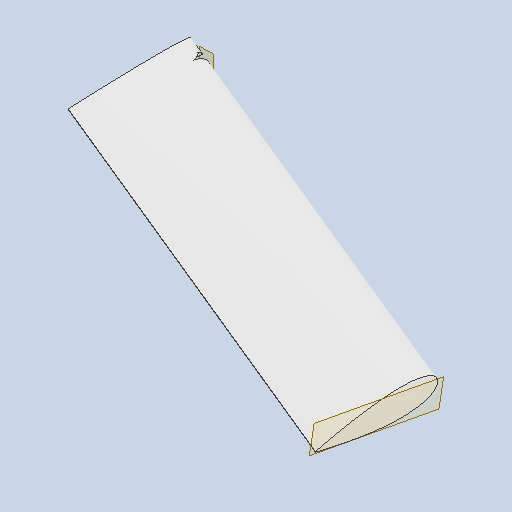
# Autodesk Inventor part: TailRight
Saved by Autodesk Inventor 2026 (Build 300175050, 175E)
## iProperties
Created: 2025-08-03
Part Number: TailRight
Material: Plastic, Opaque White
Document SubType Name: Modeling
Designer: Cupri
Density: 0.952 g/cm^3
Appearance: Smooth - White
Mass: 2293.42 g
Surface Area: 2244.69 cm^2
Volume: 2409.06 cm^3
Author: Cupri
Autodesk Inventor part; units mm, degrees
ref_plane "YZ Plane" through (0, 0, 0) normal (1, 0, 0) x (0, 1, 0)
ref_plane "XZ Plane" through (0, 0, 0) normal (0, 1, 0) x (-1, 0, 0)
ref_plane "XY Plane" through (0, 0, 0) normal (0, 0, 1) x (1, 0, 0)
sketch "Sketch1" plane through (0, 0, 0) normal (0, 0, 1) x (1, 0, 0)
  line L0 (10.5804, 9.5) -> (10.5804, 4.5) projected
  arc A0 (10.5804, 9.5) -> (10.0804, 10) centre (10.0804, 9.5) ccw projected
  line L1 (5.0804, 10) -> (10.0804, 10) projected
  line L2 (3.5804, 8.5) -> (5.0804, 10) projected
  line L3 (6.7804, 8.5) -> (3.5804, 8.5) projected
  line L4 (6.7804, 7.0485) -> (6.7804, 8.5) projected
  line L5 (3.3319, 3.6) -> (6.7804, 7.0485) projected
  line L6 (-2.1711, 3.6) -> (3.3319, 3.6) projected
  line L7 (-5.6196, 7.0485) -> (-2.1711, 3.6) projected
  line L8 (-5.6196, 8.5) -> (-5.6196, 7.0485) projected
  line L9 (-2.4196, 8.5) -> (-5.6196, 8.5) projected
  line L10 (-3.9196, 10) -> (-2.4196, 8.5) projected
  line L11 (-8.9196, 10) -> (-3.9196, 10) projected
  arc A1 (-8.9196, 10) -> (-9.4196, 9.5) centre (-8.9196, 9.5) ccw projected
  line L12 (-9.4196, 4.5) -> (-9.4196, 9.5) projected
  line L13 (-7.9196, 3) -> (-9.4196, 4.5) projected
  line L14 (-7.9196, 6.2) -> (-7.9196, 3) projected
  line L15 (-6.4681, 6.2) -> (-7.9196, 6.2) projected
  line L16 (-3.0196, 2.7515) -> (-6.4681, 6.2) projected
  line L17 (-3.0196, -2.7515) -> (-3.0196, 2.7515) projected
  line L18 (-6.4681, -6.2) -> (-3.0196, -2.7515) projected
  line L19 (-7.9196, -6.2) -> (-6.4681, -6.2) projected
  line L20 (-7.9196, -3) -> (-7.9196, -6.2) projected
  line L21 (-9.4196, -4.5) -> (-7.9196, -3) projected
  line L22 (-9.4196, -9.5) -> (-9.4196, -4.5) projected
  arc A2 (-9.4196, -9.5) -> (-8.9196, -10) centre (-8.9196, -9.5) ccw projected
  line L23 (-3.9196, -10) -> (-8.9196, -10) projected
  line L24 (-2.4196, -8.5) -> (-3.9196, -10) projected
  line L25 (-5.6196, -8.5) -> (-2.4196, -8.5) projected
  line L26 (-5.6196, -7.0485) -> (-5.6196, -8.5) projected
  line L27 (-2.1711, -3.6) -> (-5.6196, -7.0485) projected
  line L28 (3.3319, -3.6) -> (-2.1711, -3.6) projected
  line L29 (6.7804, -7.0485) -> (3.3319, -3.6) projected
  line L30 (6.7804, -8.5) -> (6.7804, -7.0485) projected
  line L31 (3.5804, -8.5) -> (6.7804, -8.5) projected
  line L32 (5.0804, -10) -> (3.5804, -8.5) projected
  line L33 (10.0804, -10) -> (5.0804, -10) projected
  arc A3 (10.0804, -10) -> (10.5804, -9.5) centre (10.0804, -9.5) ccw projected
  line L34 (10.5804, -4.5) -> (10.5804, -9.5) projected
  line L35 (9.0804, -3) -> (10.5804, -4.5) projected
  line L36 (9.0804, -6.2) -> (9.0804, -3) projected
  line L37 (7.6289, -6.2) -> (9.0804, -6.2) projected
  line L38 (4.1804, -2.7515) -> (7.6289, -6.2) projected
  line L39 (4.1804, 2.7515) -> (4.1804, -2.7515) projected
  line L40 (7.6289, 6.2) -> (4.1804, 2.7515) projected
  line L41 (9.0804, 6.2) -> (7.6289, 6.2) projected
  line L42 (9.0804, 3) -> (9.0804, 6.2) projected
  line L43 (10.5804, 4.5) -> (9.0804, 3) projected
  circle A4 centre (0.5804, 0) radius 2 projected
  line L44 (-10.125, 10.125) -> (10.125, 10.125) projected
  line L45 (-10.125, -10.125) -> (-10.125, 10.125) projected
  line L46 (385, 60.6857) -> (385, -334.3432)
  line L47 (-10.125, 10.125) -> (385, -266.5445)
  line L48 (-10.125, 10.125) -> (472.2336, 10.125) construction
  line L49 (-10.125, 10.125) -> (-18.3165, 15.8608)
  line L50 (780.125, 10.125) -> (385, -266.5445)
  ellipse E0 centre (381.713, 63.1894) end of major axis (413.2942, 37.7545) minor radius 40.5498 projected
  point P0 (0, 0)
  dimension "d0" = 35
  dimension "d1" = 10
  constraints: 10 end point, 2 point on line, 1 equal length, 1 horizontal, 1 symmetric about line, 1 vertical
  measures "d0" angle of L47 L48
  measures "d1" distance of L44.start L49.end
ref_plane "Work Plane1" through (-18.3165, 15.8608, 0) normal (-0.819152, 0.5735764, 0) x (-0.5735764, -0.819152, 0)
sketch "Sketch2" plane through (-18.3165, 15.8608, 0) normal (-0.819152, 0.5735764, 0) x (-0.5735764, -0.819152, 0)
  spline S0 degree 4 poles (3.0051, 134.0148) (3.0202, 133.9433) (3.0935, 133.5946) (3.2162, 133.0098) (3.4218, 132.0236) (3.6365, 130.9884) (3.8977, 129.7198) (4.2019, 128.23) (4.5479, 126.5185) (4.9334, 124.5915) (5.356, 122.4525) (5.8134, 120.1071) (6.3027, 117.5605) (6.8216, 114.8187) (7.367, 111.8882) (7.9363, 108.7758) (8.5263, 105.4888) (9.1344, 102.0348) (9.7573, 98.422) (10.3924, 94.6587) (11.0362, 90.7538) (11.686, 86.7164) (12.3385, 82.5558) (12.9906, 78.282) (13.6392, 73.9047) (14.2807, 69.4343) (14.912, 64.8811) (15.5296, 60.2559) (16.1298, 55.5693) (16.7091, 50.8325) (17.2636, 46.0563) (17.7897, 41.252) (18.2834, 36.4308) (18.7408, 31.6039) (19.1581, 26.7826) (19.5314, 21.9782) (19.8569, 17.2018) (20.1309, 12.4646) (20.3499, 7.7777) (20.5107, 3.1519) (20.6103, -1.4019) (20.646, -5.8731) (20.6155, -10.2512) (20.5168, -14.5261) (20.3486, -18.6878) (20.1098, -22.7266) (19.8, -26.633) (19.4191, -30.3981) (18.9678, -34.0129) (18.447, -37.4692) (17.8584, -40.7589) (17.2038, -43.8744) (16.4855, -46.8085) (15.7065, -49.5545) (14.8694, -52.1063) (13.9776, -54.4581) (13.0341, -56.6048) (12.0421, -58.5418) (11.0046, -60.2651) (9.9239, -61.7712) (8.8021, -63.0569) (7.64, -64.1189) (6.4386, -64.9533) (5.1984, -65.5542) (3.9272, -65.9158) (2.6271, -66.0345) (1.3269, -65.9158) (0.0558, -65.5542) (-1.1844, -64.9533) (-2.3858, -64.1189) (-3.5479, -63.0569) (-4.6698, -61.7712) (-5.7504, -60.2651) (-6.7879, -58.5418) (-7.7799, -56.6048) (-8.7234, -54.4581) (-9.6152, -52.1063) (-10.4523, -49.5545) (-11.2314, -46.8085) (-11.9496, -43.8744) (-12.6042, -40.7589) (-13.1929, -37.4692) (-13.7136, -34.0129) (-14.1649, -30.3981) (-14.5458, -26.633) (-14.8556, -22.7266) (-15.0944, -18.6878) (-15.2627, -14.5261) (-15.3613, -10.2512) (-15.3918, -5.8731) (-15.3562, -1.4019) (-15.2566, 3.1519) (-15.0957, 7.7777) (-14.8767, 12.4646) (-14.6027, 17.2018) (-14.2772, 21.9782) (-13.9039, 26.7826) (-13.4867, 31.6039) (-13.0292, 36.4308) (-12.5355, 41.252) (-12.0094, 46.0563) (-11.4549, 50.8325) (-10.8756, 55.5693) (-10.2754, 60.2559) (-9.6579, 64.8811) (-9.0265, 69.4343) (-8.385, 73.9047) (-7.7365, 78.282) (-7.0843, 82.5558) (-6.4318, 86.7164) (-5.782, 90.7538) (-5.1382, 94.6587) (-4.5031, 98.422) (-3.8802, 102.0348) (-3.2722, 105.4888) (-2.6821, 108.7758) (-2.1128, 111.8882) (-1.5674, 114.8187) (-1.0485, 117.5605) (-0.5592, 120.1071) (-0.1018, 122.4525) (0.3208, 124.5915) (0.7063, 126.5185) (1.0523, 128.23) (1.3565, 129.7198) (1.6177, 130.9884) (1.8324, 132.0236) (2.038, 133.0098) (2.1607, 133.5946) (2.234, 133.9433) (2.2491, 134.0148) knots 0 0 0 0 0 0.006257 0.009939 0.014222 0.019019 0.024272 0.029938 0.03598 0.04237 0.04908 0.05609 0.063377 0.070923 0.07871 0.086722 0.094944 0.10336 0.111956 0.120718 0.129633 0.138688 0.147869 0.157166 0.166564 0.176052 0.185618 0.19525 0.204936 0.214665 0.224425 0.234204 0.243991 0.253774 0.263543 0.273285 0.282989 0.292645 0.30224 0.311765 0.321208 0.330557 0.339803 0.348934 0.357939 0.366808 0.37553 0.384093 0.392488 0.400704 0.40873 0.416554 0.424168 0.431561 0.438722 0.445644 0.452318 0.45874 0.464908 0.470825 0.476503 0.481964 0.487245 0.492398 0.497475 0.502525 0.507602 0.512755 0.518036 0.523497 0.529175 0.535092 0.54126 0.547682 0.554356 0.561278 0.568439 0.575832 0.583446 0.59127 0.599296 0.607512 0.615907 0.62447 0.633192 0.642061 0.651066 0.660197 0.669443 0.678792 0.688235 0.69776 0.707355 0.717011 0.726715 0.736457 0.746226 0.756009 0.765796 0.775575 0.785335 0.795064 0.80475 0.814382 0.823948 0.833436 0.842834 0.852131 0.861312 0.870367 0.879282 0.888044 0.89664 0.905056 0.913278 0.92129 0.929077 0.936623 0.94391 0.95092 0.95763 0.96402 0.970062 0.975728 0.980981 0.985778 0.990061 0.993743 1 1 1 1 1
  line L0 (3.0051, 134.0148) -> (2.2491, 134.0148)
  point P0 (3.0297, 133.898)
  point P1 (3.1032, 133.5479)
  point P2 (3.2252, 132.9654)
  point P3 (3.3949, 132.1518)
  point P4 (3.6112, 131.1089)
  point P5 (3.8727, 129.8393)
  point P6 (4.1776, 128.3459)
  point P7 (4.5242, 126.6322)
  point P8 (4.9103, 124.7022)
  point P9 (5.3336, 122.5604)
  point P10 (5.7916, 120.2117)
  point P11 (6.2818, 117.6618)
  point P12 (6.8014, 114.9165)
  point P13 (7.3476, 111.9822)
  point P14 (7.9177, 108.8658)
  point P15 (8.5086, 105.5747)
  point P16 (9.1175, 102.1163)
  point P17 (9.7413, 98.499)
  point P18 (10.3772, 94.731)
  point P19 (11.0219, 90.8212)
  point P20 (11.6725, 86.7788)
  point P21 (12.3259, 82.6131)
  point P22 (12.9788, 78.3339)
  point P23 (13.6281, 73.9512)
  point P24 (14.2704, 69.4753)
  point P25 (14.9023, 64.9165)
  point P26 (15.5204, 60.2855)
  point P27 (16.1211, 55.5932)
  point P28 (16.7008, 50.8505)
  point P29 (17.2557, 46.0684)
  point P30 (17.7819, 41.2582)
  point P31 (18.2757, 36.4311)
  point P32 (18.7331, 31.5984)
  point P33 (19.1502, 26.7713)
  point P34 (19.5231, 21.9611)
  point P35 (19.8481, 17.1791)
  point P36 (20.1214, 12.4363)
  point P37 (20.3397, 7.744)
  point P38 (20.4995, 3.1131)
  point P39 (20.5979, -1.4457)
  point P40 (20.6322, -5.9217)
  point P41 (20.6001, -10.3044)
  point P42 (20.4997, -14.5836)
  point P43 (20.3295, -18.7493)
  point P44 (20.0885, -22.7917)
  point P45 (19.7763, -26.7015)
  point P46 (19.3928, -30.4695)
  point P47 (18.9385, -34.0868)
  point P48 (18.4146, -37.5451)
  point P49 (17.8225, -40.8363)
  point P50 (17.1641, -43.9527)
  point P51 (16.4418, -46.8869)
  point P52 (15.6582, -49.6323)
  point P53 (14.8164, -52.1822)
  point P54 (13.9195, -54.5308)
  point P55 (12.9708, -56.6727)
  point P56 (11.9739, -58.6027)
  point P57 (10.9319, -60.3164)
  point P58 (9.8483, -61.8098)
  point P59 (8.7261, -63.0794)
  point P60 (7.5683, -64.1223)
  point P61 (6.3774, -64.9359)
  point P62 (5.1558, -65.5184)
  point P63 (3.9052, -65.8685)
  point P64 (2.6271, -65.9852)
  point P65 (1.349, -65.8685)
  point P66 (0.0984, -65.5184)
  point P67 (-1.1232, -64.9359)
  point P68 (-2.3141, -64.1223)
  point P69 (-3.4719, -63.0794)
  point P70 (-4.5941, -61.8098)
  point P71 (-5.6777, -60.3164)
  point P72 (-6.7197, -58.6027)
  point P73 (-7.7167, -56.6727)
  point P74 (-8.6653, -54.5308)
  point P75 (-9.5622, -52.1822)
  point P76 (-10.404, -49.6323)
  point P77 (-11.1876, -46.8869)
  point P78 (-11.9099, -43.9527)
  point P79 (-12.5683, -40.8363)
  point P80 (-13.1604, -37.5451)
  point P81 (-13.6844, -34.0868)
  point P82 (-14.1386, -30.4695)
  point P83 (-14.5221, -26.7015)
  point P84 (-14.8344, -22.7917)
  point P85 (-15.0753, -18.7493)
  point P86 (-15.2456, -14.5836)
  point P87 (-15.346, -10.3044)
  point P88 (-15.3781, -5.9217)
  point P89 (-15.3438, -1.4457)
  point P90 (-15.2453, 3.1131)
  point P91 (-15.0855, 7.744)
  point P92 (-14.8673, 12.4363)
  point P93 (-14.5939, 17.1791)
  point P94 (-14.2689, 21.9611)
  point P95 (-13.896, 26.7713)
  point P96 (-13.4789, 31.5984)
  point P97 (-13.0215, 36.4311)
  point P98 (-12.5277, 41.2582)
  point P99 (-12.0015, 46.0684)
  point P100 (-11.4466, 50.8505)
  point P101 (-10.867, 55.5932)
  point P102 (-10.2663, 60.2855)
  point P103 (-9.6481, 64.9165)
  point P104 (-9.0162, 69.4753)
  point P105 (-8.3739, 73.9512)
  point P106 (-7.7247, 78.3339)
  point P107 (-7.0717, 82.6131)
  point P108 (-6.4184, 86.7788)
  point P109 (-5.7678, 90.8212)
  point P110 (-5.123, 94.731)
  point P111 (-4.4872, 98.499)
  point P112 (-3.8633, 102.1163)
  point P113 (-3.2544, 105.5747)
  point P114 (-2.6635, 108.8658)
  point P115 (-2.0934, 111.9822)
  point P116 (-1.5472, 114.9165)
  point P117 (-1.0276, 117.6618)
  point P118 (-0.5375, 120.2117)
  point P119 (-0.0794, 122.5604)
  point P120 (0.3438, 124.7022)
  point P121 (0.7299, 126.6322)
  point P122 (1.0765, 128.3459)
  point P123 (1.3815, 129.8393)
  point P124 (1.643, 131.1089)
  point P125 (1.8592, 132.1518)
  point P126 (2.0289, 132.9654)
  point P127 (2.151, 133.5479)
  point P128 (2.2245, 133.898)
  constraints: 2 end point, 1 horizontal, 131 other
sweep "Sweep1" add profiles "Sketch2" path "Sketch1" path curves L49 L47 L50
ref_plane "Work Plane2" through (385, -270.213, 134.0148) normal (1, 0, 0) x (0, -0.1835872, -0.9830034)
split "Split1" plane through (385, -270.213, 134.0148) removes the side toward (1, 0, 0)
ref_plane "Work Plane3" through (-1.9691, -9.3576, -74.7284) normal (0, 0, 1) x (0.9998865, 0.015069, 0)
sketch "Sketch3" plane through (-1.9691, -9.3576, -74.7284) normal (0, 0, 1) x (0.9998865, 0.015069, 0)
  line L0 (12.8322, 18.6663) -> (12.7568, 13.6669) construction
  arc A0 (12.8322, 18.6663) -> (12.3398, 19.1738) centre (12.3322, 18.6738) ccw construction
  line L1 (7.3403, 19.2491) -> (12.3398, 19.1738) construction
  line L2 (5.8179, 17.7719) -> (7.3403, 19.2491) construction
  line L3 (9.0175, 17.7237) -> (5.8179, 17.7719) construction
  line L4 (8.9957, 16.2724) -> (9.0175, 17.7237) construction
  line L5 (5.4956, 12.8762) -> (8.9957, 16.2724) construction
  line L6 (-0.0067, 12.9591) -> (5.4956, 12.8762) construction
  line L7 (-3.4029, 16.4592) -> (-0.0067, 12.9591) construction
  line L8 (-3.381, 17.9105) -> (-3.4029, 16.4592) construction
  line L9 (-0.1814, 17.8623) -> (-3.381, 17.9105) construction
  line L10 (-1.6586, 19.3847) -> (-0.1814, 17.8623) construction
  line L11 (-6.6581, 19.4601) -> (-1.6586, 19.3847) construction
  arc A1 (-6.6581, 19.4601) -> (-7.1655, 18.9677) centre (-6.6656, 18.9602) ccw construction
  line L12 (-7.2409, 13.9683) -> (-7.1655, 18.9677) construction
  line L13 (-5.7637, 12.4458) -> (-7.2409, 13.9683) construction
  line L14 (-5.7154, 15.6455) -> (-5.7637, 12.4458) construction
  line L15 (-4.2641, 15.6236) -> (-5.7154, 15.6455) construction
  line L16 (-0.868, 12.1235) -> (-4.2641, 15.6236) construction
  line L17 (-0.9509, 6.6212) -> (-0.868, 12.1235) construction
  line L18 (-4.451, 3.225) -> (-0.9509, 6.6212) construction
  line L19 (-5.9023, 3.2469) -> (-4.451, 3.225) construction
  line L20 (-5.8541, 6.4465) -> (-5.9023, 3.2469) construction
  line L21 (-7.3765, 4.9693) -> (-5.8541, 6.4465) construction
  line L22 (-7.4519, -0.0302) -> (-7.3765, 4.9693) construction
  arc A2 (-7.4519, -0.0302) -> (-6.9594, -0.5376) centre (-6.9519, -0.0377) ccw construction
  line L23 (-1.96, -0.613) -> (-6.9594, -0.5376) construction
  line L24 (-0.4376, 0.8642) -> (-1.96, -0.613) construction
  line L25 (-3.6372, 0.9125) -> (-0.4376, 0.8642) construction
  line L26 (-3.6153, 2.3638) -> (-3.6372, 0.9125) construction
  line L27 (-0.1152, 5.7599) -> (-3.6153, 2.3638) construction
  line L28 (5.3871, 5.677) -> (-0.1152, 5.7599) construction
  line L29 (8.7832, 2.1769) -> (5.3871, 5.677) construction
  line L30 (8.7614, 0.7256) -> (8.7832, 2.1769) construction
  line L31 (5.5617, 0.7738) -> (8.7614, 0.7256) construction
  line L32 (7.039, -0.7486) -> (5.5617, 0.7738) construction
  line L33 (12.0384, -0.8239) -> (7.039, -0.7486) construction
  arc A3 (12.0384, -0.8239) -> (12.5459, -0.3315) centre (12.0459, -0.324) ccw construction
  line L34 (12.6212, 4.6679) -> (12.5459, -0.3315) construction
  line L35 (11.144, 6.1903) -> (12.6212, 4.6679) construction
  line L36 (11.0958, 2.9907) -> (11.144, 6.1903) construction
  line L37 (9.6445, 3.0126) -> (11.0958, 2.9907) construction
  line L38 (6.2483, 6.5127) -> (9.6445, 3.0126) construction
  line L39 (6.3312, 12.015) -> (6.2483, 6.5127) construction
  line L40 (9.8313, 15.4112) -> (6.3312, 12.015) construction
  line L41 (11.2826, 15.3893) -> (9.8313, 15.4112) construction
  line L42 (11.2344, 12.1896) -> (11.2826, 15.3893) construction
  line L43 (12.7568, 13.6669) -> (11.2344, 12.1896) construction
  circle A4 centre (2.6902, 9.3181) radius 2 construction
  line L44 (-7.5598, -0.9319) -> (12.9402, -0.9319)
  line L45 (12.9402, -0.9319) -> (12.9402, 19.5681)
  line L46 (12.9402, 19.5681) -> (-7.5598, 19.5681)
  line L47 (-7.5598, 19.5681) -> (-7.5598, -0.9319)
  line L48 (-7.5598, -0.9319) -> (12.9402, 19.5681) construction
  line L49 (12.9402, -0.9319) -> (-7.5598, 19.5681) construction
  line L50 (5.4402, 19.5681) -> (-0.0598, 19.5681) construction
  line L51 (-0.0598, 19.5681) -> (-0.0598, 14.0681)
  line L52 (-0.0598, 14.0681) -> (5.4402, 14.0681)
  line L53 (5.4402, 14.0681) -> (5.4402, 19.5681)
  line L54 (12.9402, 9.3181) -> (-7.5598, 9.3181) construction
  line L55 (-0.0598, -0.9319) -> (-0.0598, 4.5681)
  line L56 (-0.0598, 4.5681) -> (5.4402, 4.5681)
  line L57 (5.4402, 4.5681) -> (5.4402, -0.9319)
  point P0 (2.1098, 9.3268)
  point P1 (-0.0598, -0.9319)
  point P2 (5.4402, -0.9319)
  dimension "d5" = 20.5
  dimension "d6" = 20.5
  dimension "d7" = 5.5
  dimension "d8" = 5.5
  dimension "d9" = 13
  constraints: 28 end point, 4 midpoint, 4 parallel, 4 symmetric about line, 2 horizontal, 2 perpendicular, 1 point on line
  measures "d5" distance of L46.end L45.end
  measures "d6" distance of L45.end L44.end
  measures "d7" distance of L52.end L51.end
  measures "d8" distance of L51.end L50.end
  measures "d9" distance between parallel lines of L45 L51
extrude "Extrusion1" cut sketch "Sketch3" along normal blind 90 contours L47 L46 L51 L52 L53 L45 L44 L57 L56 L55
sketch "Sketch4" plane through (-19.8234, 13.7088, 34.0148) normal (-0.819152, 0.5735764, 0) x (0.1182491, 0.1688772, 0.9785181)
  circle A0 centre (-75.1353, 17.1475) radius 2.75
  point P0 (-33.2551, 7.1501)
  dimension "d12" = 5.5
  constraints: 1 centre point
  measures "d12" diameter of A0
hole "Hole1" at (-19.0839, 14.7648, -43.0416) direction (0.819152, -0.5735764, 0) diameter 5.3 depth 28 counterbore diameter 8.5 counterbore depth 8
body "Solid1"
